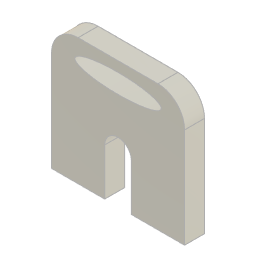
GC Port Clip (Autodesk Fusion 360 design; units mm, degrees)
Autodesk Fusion 360 part; units mm, degrees
note: some values were not read from the file. Set by a fixed rule: which sketch regions a step uses.
sketch "Sketch1" plane through (0, 0, 0) normal (0, 0, 1) x (1, 0, 0)
  line L0 (10, 1.5) -> (-10, 1.5)
  line L1 (-10, 1.5) -> (-10, -1.5)
  line L2 (-10, -1.5) -> (10, -1.5)
  line L3 (10, -1.5) -> (10, 1.5)
  dimension "d1" = 20
  dimension "d2" = 3
  constraint horizontal L0
  constraint perpendicular L0 L1
  constraint parallel L0 L2
  constraint parallel L1 L3
  measures "d1" distance of L1.end L2.end
  measures "d2" distance of L0.end L1.end
extrude "Extrude1" add sketch "Sketch1" along normal blind 19
sketch "Sketch2" plane through (0, 1.5, 0) normal (0, 1, 0) x (-1, 0, 0)
  line L0 (-10, 0) -> (10, 0)
  line L1 (10, 0) -> (10, 19)
  line L2 (10, 19) -> (-10, 19)
  line L3 (-10, 19) -> (-10, 0)
  line L4 (0, 9.05) -> (0, 9.05)
  line L5 (-2, 7.05) -> (-2, 0)
  line L6 (2, 7.05) -> (2, 0)
  arc A0 (0, 9.05) -> (-2, 7.05) centre (0, 7.05) ccw
  arc A1 (2, 7.05) -> (0, 9.05) centre (0, 7.05) ccw
  point P0 (0, 9.05)
  dimension "d9" = 2
  constraint coincident L0 L5.end
  constraint perpendicular L0 L5
  constraint coincident L0 L6.end
  constraint perpendicular L0 L6
  constraint tangent L5 A0
  constraint tangent L6 A1
  constraint equal A0 A1
  measures "d9" radius of A0
extrude "Extrude2" cut sketch "Sketch2" against normal blind 3 contours L0 L5 L6 A0 A1
fillet "Fillet1" radius 4 2 edges at (10, 0, 19) (-10, 0, 19)
sketch "Sketch3" plane through (0, 1.5, 0) normal (0, 1, 0) x (-1, 0, 0)
  arc A0 (10, 15) -> (6, 19) centre (6, 15) ccw
  line L0 (6, 19) -> (-6, 19)
  arc A1 (-6, 19) -> (-10, 15) centre (-6, 15) ccw
  line L1 (-10, 15) -> (-10, 0)
  line L2 (-10, 0) -> (-2, 0)
  line L3 (-2, 0) -> (-2, 7.05)
  arc A2 (2, 7.05) -> (-2, 7.05) centre (0, 7.05) ccw
  line L4 (2, 7.05) -> (2, 0)
  line L5 (2, 0) -> (10, 0)
  line L6 (10, 0) -> (10, 15)
  line L7 (0, 19) -> (0, 13.1)
  line L8 (0, 19) -> (0, 17.5)
  line L9 (0, 13.1) -> (0, 14.6)
  ellipse E0 centre (0, 16.05) end of major axis (0, 17.5) minor radius 6.5
  line L10 (0, 14.6) -> (0, 17.5)
  line L11 (6.5, 16.05) -> (-6.5, 16.05)
  dimension "d14" = 5.9
  dimension "d15" = 1.5
  dimension "d16" = 1.5
  dimension "d17" = 13
  constraint midpoint L0 L7.start
  constraint perpendicular L0 L7
  constraint perpendicular L0 L8
  constraint parallel L7 L9
  constraint midpoint L7 E0.centre
  constraint coincident L9.end E0
  constraint coincident E0 L11.start
  constraint coincident E0 L11.end
  measures "d14" distance of L7.start L7.end
  measures "d15" distance of L7.start L8.end
  measures "d16" distance of L7.end L9.end
extrude "Extrude3" cut sketch "Sketch3" against normal blind 3 contours L7 E0 L10 L11 | L7 E0 L10 L11 | L7 E0 L10 L11 | L7 E0 L10 L11
